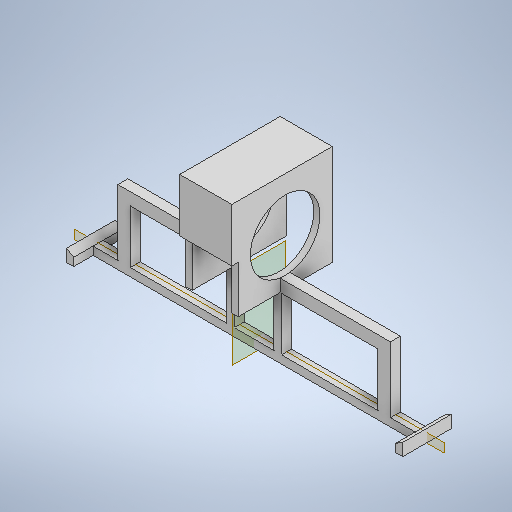
# Autodesk Inventor part: 2024_09_24_Holder_Power_sensor
Saved by Autodesk Inventor 2025.1 (Build 291241000, 241)
## iProperties
Created: 2024-08-23
Part Number: 2024_09_24_Holder_Power_sensor
Material: Generisch
Document SubType Name: Modeling
Designer: to86hug
Density: 1 g/cm^3
Appearance: Vorgabe
Author: to86hug
Autodesk Inventor part; units mm, degrees
ref_plane "YZ Plane" through (0, 0, 0) normal (1, 0, 0) x (0, 1, 0)
ref_plane "XZ Plane" through (0, 0, 0) normal (0, 1, 0) x (-1, 0, 0)
ref_plane "XY Plane" through (0, 0, 0) normal (0, 0, 1) x (1, 0, 0)
sketch "Skizze1" plane through (0, 0, 0) normal (0, 0, 1) x (1, 0, 0)
  line L0 (-68.016, 1.808) -> (67.584, 1.808)
  line L1 (67.584, 1.808) -> (67.584, -2.192)
  line L2 (67.584, -2.192) -> (-68.016, -2.192)
  line L3 (-68.016, -2.192) -> (-68.016, 1.808)
  line L4 (-68.016, 1.808) -> (67.584, -2.192) construction
  line L5 (67.584, 1.808) -> (-68.016, -2.192) construction
  point P0 (0, 0)
  point P1 (-0.216, -0.192)
  point P2 (-0.216, -0.192)
  dimension "d0" = 135.6
  dimension "d1" = 4
  constraints: 12 end point, 2 midpoint, 2 parallel, 1 horizontal, 1 perpendicular
  measures "d0" distance of L0.start L0.end
  measures "d1" distance of L0.end L1.end
extrude "Extrusion1" add sketch "Skizze1" along normal mid plane 3.25
ref_plane "Arbeitsebene1" through (-68.016, -0.192, 1.625) normal (0, -1, 0) x (1, 0, 0)
sketch "Skizze2" plane through (-68.016, -0.192, 1.625) normal (0, -1, 0) x (1, 0, 0)
  line L0 (0, -3.25) -> (0, 0) projected
  line L1 (0, -3.25) -> (135.6, -3.25) projected
  line L2 (0, 0) -> (2.85, 0)
  line L3 (2.85, 0) -> (2.85, -3.25)
  line L4 (2.85, -3.25) -> (0, -3.25)
  line L5 (0, -3.25) -> (0, 0)
  line L6 (0, 0) -> (0, 1.75)
  line L7 (0, 1.75) -> (2.85, 0)
  line L8 (135.6, -3.25) -> (135.6, 0) projected
  line L9 (135.6, 0) -> (132.75, 0)
  line L10 (132.75, 0) -> (132.75, -3.25)
  line L11 (132.75, -3.25) -> (135.6, -3.25)
  line L12 (135.6, -3.25) -> (135.6, 0)
  line L13 (135.6, 0) -> (135.6, 1.75)
  line L14 (135.6, 1.75) -> (132.75, 0)
  point P0 (68.016, -1.625)
  dimension "d4" = 2.85
  dimension "d5" = 1.75
  dimension "d6" = 2.85
  constraints: 24 end point, 4 parallel, 2 horizontal, 2 perpendicular, 2 point on line, 2 vertical
  measures "d4" distance of L3.end L4.end
  measures "d5" distance of L0.end L6.end
  measures "d6" distance of L11.end L10.end
extrude "Extrusion2" add sketch "Skizze2" along normal mid plane 19.7
sketch "Skizze7" plane through (0, 0, 1.625) normal (0, 0, 1) x (1, 0, 0)
  line L0 (-65.166, 9.658) -> (-65.166, 1.808) projected
  line L1 (-65.166, 1.808) -> (-55.166, 1.808)
  line L2 (64.734, 1.808) -> (-65.166, 1.808) projected
  line L3 (64.734, -2.192) -> (-65.166, -2.192) projected
  line L4 (64.734, -2.192) -> (54.734, -2.192)
  line L5 (-55.166, 1.808) -> (54.734, 1.808)
  line L6 (54.734, 1.808) -> (54.734, -2.192)
  line L7 (54.734, -2.192) -> (-55.166, -2.192)
  line L8 (-55.166, -2.192) -> (-55.166, 1.808)
  point P0 (0, 0)
  dimension "d27" = 10
  dimension "d28" = 10
  constraints: 12 end point, 2 parallel, 2 point on line, 1 horizontal, 1 perpendicular
  measures "d27" distance of L0.end L1.end
  measures "d28" distance of L3.start L4.end
extrude "Extrusion7" add sketch "Skizze7" along normal blind 26.5
sketch "Skizze8" plane through (0, 0, 1.625) normal (0, 0, 1) x (1, 0, 0)
  line L0 (-65.166, 1.808) -> (-50.166, 1.808)
  line L1 (-65.166, 1.808) -> (64.734, 1.808) projected
  line L2 (64.734, -2.192) -> (-65.166, -2.192) projected
  line L3 (64.734, -2.192) -> (49.734, -2.192)
  line L4 (-50.166, 1.808) -> (49.734, 1.808)
  line L5 (49.734, 1.808) -> (49.734, -2.192)
  line L6 (49.734, -2.192) -> (-50.166, -2.192)
  line L7 (-50.166, -2.192) -> (-50.166, 1.808)
  point P0 (0, 0)
  dimension "d31" = 15
  dimension "d32" = 15
  constraints: 12 end point, 2 parallel, 2 point on line, 1 horizontal, 1 perpendicular
  measures "d31" distance of L0.start L0.end
  measures "d32" distance of L2.start L3.end
extrude "Extrusion8" cut sketch "Skizze8" along normal blind 21.5
ref_plane "Arbeitsebene2" through (-0.216, -10.042, -1.625) normal (-1, 0, 0) x (0, 0, 1)
sketch "Skizze9" plane through (-0.216, -10.042, -1.625) normal (-1, 0, 0) x (0, 0, 1)
  line L0 (24.75, 11.85) -> (29.75, 11.85)
  line L1 (29.75, 11.85) -> (29.75, 7.85)
  line L2 (29.75, 7.85) -> (24.75, 7.85)
  line L3 (24.75, 7.85) -> (24.75, 11.85)
  point P0 (1.625, 10.042)
  constraints: 8 end point, 2 parallel, 1 horizontal, 1 perpendicular
extrude "Extrusion9" cut sketch "Skizze9" along normal mid plane 14
sketch "Skizze17" plane through (-0.216, -10.042, -1.625) normal (-1, 0, 0) x (0, 0, 1)
  line L0 (24.75, 11.85) -> (24.75, 28.85) projected
  line L1 (62.75, -9.15) -> (62.75, 28.85) projected
  line L2 (24.75, 28.85) -> (62.75, 28.85)
  line L3 (62.75, 28.85) -> (62.75, -9.15)
  line L4 (62.75, -9.15) -> (24.75, -9.15)
  line L5 (24.75, -9.15) -> (24.75, 28.85)
  circle A0 centre (43.75, 9.85) radius 14
  point P0 (1.625, 10.042)
  constraints: 8 end point, 2 parallel, 1 centre point, 1 horizontal, 1 perpendicular
extrude "Extrusion19" add sketch "Skizze17" along normal mid plane 21
sketch "Skizze19" plane through (-0.216, -10.042, -1.625) normal (-1, 0, 0) x (0, 0, 1)
  line L0 (24.75, 28.85) -> (24.75, 11.85) projected
  line L1 (24.75, -9.15) -> (62.75, -9.15) projected
  line L2 (24.75, 28.85) -> (62.75, 28.85)
  line L3 (62.75, 28.85) -> (62.75, -9.15)
  line L4 (62.75, -9.15) -> (24.75, -9.15)
  line L5 (24.75, -9.15) -> (24.75, 28.85)
  point P0 (1.625, 10.042)
  point P1 (24.75, 11.85)
  constraints: 8 end point, 2 parallel, 1 horizontal, 1 perpendicular
extrude "Extrusion20" cut sketch "Skizze19" along normal mid plane 16
sketch "Skizze20" plane through (10.284, -19.192, 61.125) normal (0, 0, 1) x (1, 0, 0)
  line L0 (0, 38) -> (0, 0) projected
  line L1 (0, 38) -> (-21, 38)
  line L2 (-21, 38) -> (-21, 0)
  line L3 (-21, 0) -> (0, 0)
  line L4 (0, 0) -> (0, 38)
  point P0 (-10.284, 19.192)
  constraints: 8 end point, 2 parallel, 1 horizontal, 1 perpendicular
extrude "Extrusion21" add sketch "Skizze20" along normal blind 2.5
sketch "Skizze21" plane through (7.784, -19.192, 23.125) normal (0, -1, 0) x (1, 0, 0)
  line L0 (-18.5, 5) -> (-18.5, 33) projected
  line L1 (2.5, 40.5) -> (-18.5, 40.5)
  line L2 (-18.5, 40.5) -> (-18.5, 19)
  line L3 (-18.5, 19) -> (2.5, 19)
  line L4 (2.5, 19) -> (2.5, 40.5)
  point P0 (-7.784, -23.125)
  constraints: 8 end point, 2 parallel, 1 horizontal, 1 midpoint, 1 perpendicular
extrude "Extrusion22" add sketch "Skizze21" along normal blind 2.5
sketch "Skizze22" plane through (0, 0, 23.125) normal (0, 0, -1) x (-1, 0, 0)
  line L0 (-54.734, 1.808) -> (-10.284, 1.808) projected
  line L1 (-10.284, 1.808) -> (-7.784, 1.808)
  line L2 (-7.784, 18.808) -> (-7.784, -19.192) projected
  line L3 (-10.284, 1.808) -> (-7.784, 1.808) construction
  line L4 (-10.284, -2.192) -> (-54.734, -2.192) projected
  line L5 (-7.784, 1.808) -> (-10.784, 1.808)
  line L6 (-10.784, 1.808) -> (-10.784, -2.192)
  line L7 (-10.784, -2.192) -> (-7.784, -2.192)
  line L8 (-7.784, -2.192) -> (-7.784, 1.808)
  line L9 (10.716, 18.808) -> (10.716, -21.692) projected
  line L10 (10.716, -2.192) -> (8.216, -2.192)
  line L11 (8.216, -2.192) -> (11.216, -2.192)
  line L12 (11.216, -2.192) -> (11.216, 1.808)
  line L13 (11.216, 1.808) -> (8.216, 1.808)
  line L14 (8.216, 1.808) -> (8.216, -2.192)
  point P0 (0, 0)
  dimension "d79" = 2.5
  dimension "d80" = 0
  dimension "d81" = 3
  dimension "d82" = 2.5
  dimension "d83" = 3
  constraints: 22 end point, 4 horizontal, 4 parallel, 3 perpendicular, 2 point on line, 1 collinear
  measures "d79" distance of L0.end L1.end
  measures "d80" distance between parallel lines of L1 L3
  measures "d81" distance of L7.end L6.end
  measures "d82" distance of L10.start L10.end
  measures "d83" distance of L13.end L12.end
extrude "Extrusion23" add sketch "Skizze22" along normal up to surface (24.75 mm away)
